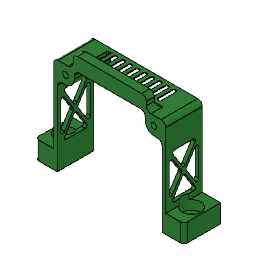
RM Carriage Setup (Defensemen) (Autodesk Fusion 360 archive; units mm, degrees)
design "LGR RM Front Holder (Defensemen)"
Autodesk Fusion 360 part; units mm, degrees
(part 1 of 2)
sketch "Sketch1" plane through (0, 0, 0) normal (0, 0, 1) x (1, 0, 0)
  line L0 (28.55, 26.275) -> (30.55, 26.275)
  line L1 (30.55, 26.275) -> (30.55, -26.275)
  line L2 (30.55, -26.275) -> (28.55, -26.275)
  line L3 (28.55, -26.275) -> (28.55, 26.275)
  line L4 (-28.55, -26.275) -> (-30.55, -26.275)
  line L5 (-28.55, 26.275) -> (-28.55, -26.275)
  line L6 (-30.55, -26.275) -> (-30.55, 26.275)
  line L7 (-30.55, 26.275) -> (-28.55, 26.275)
  line L8 (-30.55, 26.275) -> (30.55, 26.275)
  line L9 (30.55, 26.275) -> (30.55, 28.275)
  line L10 (30.55, 28.275) -> (-30.55, 28.275)
  line L11 (-30.55, 28.275) -> (-30.55, 26.275)
  dimension "d1" = 2
  dimension "d2" = 52.55
  dimension "d4" = 26.275
  dimension "d5" = 2
  dimension "d6" = 52.55
  dimension "d7" = 57.1
  dimension "d8" = 28.55
  dimension "d9" = 2
  constraint horizontal L0
  constraint vertical L1
  constraint horizontal L2
  constraint vertical L3
  constraint horizontal L7
  constraint vertical L5
  constraint horizontal L4
  constraint vertical L6
  constraint horizontal L2.end L4.start
  constraint horizontal L8
  constraint vertical L9
  constraint horizontal L10
  constraint vertical L11
  constraint vertical L0.end L9.end
  measures "d1" distance of L1 L3
  measures "d2" distance of L0 L2
  measures "d4" distance of origin L0
  measures "d5" distance of L5 L6
  measures "d6" distance of L4 L7
  measures "d7" distance of L3 L5
  measures "d8" distance of origin L5
  measures "d9" distance of L8 L10
extrude "Extrude1" add sketch "Sketch1" along normal blind 20
sketch "Sketch2" plane through (0, 0, 20) normal (0, 0, 1) x (-1, 0, 0)
  line L0 (-30.55, 26.275) -> (-30.55, -28.275)
  line L1 (-30.55, -28.275) -> (30.55, -28.275)
  line L2 (30.55, -28.275) -> (30.55, 26.275)
  line L3 (30.55, 26.275) -> (28.55, 26.275)
  line L4 (28.55, 26.275) -> (28.55, -26.275)
  line L5 (28.55, -26.275) -> (-28.55, -26.275)
  line L6 (-28.55, -26.275) -> (-28.55, 26.275)
  line L7 (-28.55, 26.275) -> (-30.55, 26.275)
  line L8 (-30.55, 26.275) -> (-40.55, 26.275)
  line L9 (-40.55, 26.275) -> (-40.55, 16.275)
  line L10 (-40.55, 16.275) -> (-30.55, 16.275)
  line L11 (-30.55, 16.275) -> (-30.55, 26.275)
  line L12 (30.55, 26.275) -> (40.55, 26.275)
  line L13 (40.55, 26.275) -> (40.55, 16.275)
  line L14 (40.55, 16.275) -> (30.55, 16.275)
  line L15 (30.55, 16.275) -> (30.55, 26.275)
  dimension "d12" = 10
  dimension "d13" = 10
  dimension "d14" = 10
  dimension "d15" = 10
  constraint horizontal L8
  constraint vertical L9
  constraint horizontal L10
  constraint vertical L11
  constraint coincident L0.start L7.end
  constraint horizontal L12
  constraint vertical L13
  constraint horizontal L14
  constraint vertical L15
  constraint coincident L2.end L3.start
  measures "d12" distance of L8 L10
  measures "d13" distance of L9 L11
  measures "d14" distance of L12 L14
  measures "d15" distance of L13 L15
extrude "Extrude2" add sketch "Sketch2" against normal blind 20 contours L0 L8 L9 L10 L11 | L2 L12 L13 L14 L15
fillet "Fillet1" radius 2 2 edges at (40.55, -21.275, 0) (-40.55, -21.275, 0)
sketch "Sketch3" plane through (0, -16.275, 0) normal (0, 1, 0) x (-1, 0, 0)
  arc A0 (38.55, 0) -> (40.55, 2) centre (38.55, 2) ccw
  line L0 (40.55, 2) -> (40.55, 20)
  line L1 (40.55, 20) -> (30.55, 20)
  line L2 (30.55, 20) -> (30.55, 0)
  line L3 (30.55, 0) -> (38.55, 0)
  point P0 (34.75, 10)
  point P1 (-34.75, 10)
  dimension "d20" = 5.8
  dimension "d21" = 10
  dimension "d22" = 69.5
  constraint horizontal P0 P1
  measures "d20" distance of L0 P0
  measures "d21" distance of L3 P0
  measures "d22" distance of P0 P1
hole "Hole1" at (-34.75, -16.275, 10) at (34.75, -16.275, 10) direction (0, -1, 0) diameter 5.3 end through all counterbore diameter 10 counterbore depth 5
sketch "Sketch4" plane through (0, -16.275, 0) normal (0, 1, 0) x (-1, 0, 0)
  arc A0 (30.55, 7.2871) -> (30.55, 12.7129) centre (34.75, 10) ccw
  line L0 (30.55, 7.2871) -> (30.55, 0)
  line L1 (30.55, 0) -> (38.55, 0)
  arc A1 (38.55, 0) -> (40.55, 2) centre (38.55, 2) ccw
  line L2 (40.55, 2) -> (40.55, 20)
  line L3 (40.55, 20) -> (30.55, 20)
  line L4 (30.55, 20) -> (30.55, 12.7129)
  circle A2 centre (34.75, 10) radius 5
  circle A3 centre (-34.75, 10) radius 5
  dimension "d28" = 10
  dimension "d29" = 69.5
  constraint concentric A0 A2
  constraint coincident A0.end A2
  constraint horizontal A0.centre A3.centre
  measures "d28" diameter of A3
  measures "d29" distance of A0.centre A3.centre
extrude "Extrude3" cut sketch "Sketch4" along normal blind 7 contours A0 A2 | A3
sketch "Sketch5" plane through (0, 28.275, 0) normal (0, 1, 0) x (-1, 0, 0)
  line L0 (-30.55, 0) -> (30.55, 0)
  line L1 (30.55, 0) -> (30.55, 20)
  line L2 (30.55, 20) -> (-30.55, 20)
  line L3 (-30.55, 20) -> (-30.55, 0)
  line L4 (-20, 20) -> (20, 20)
  line L5 (20, 20) -> (20, 0)
  line L6 (20, 0) -> (-20, 0)
  line L7 (-20, 0) -> (-20, 20)
  dimension "d32" = 40
  dimension "d96" = 20
  constraint horizontal L4
  constraint vertical L5
  constraint horizontal L6
  constraint vertical L7
  constraint coincident L0 L5.end
  constraint coincident L2 L4.start
  measures "d32" distance of L5 L7
  measures "d96" distance of origin L7
extrude "Extrude4" add sketch "Sketch5" along normal blind 10 contours L0 L2 L4 L5 L6 L7
sketch "Sketch6" plane through (0, 0, 0) normal (0, 0, -1) x (1, 0, 0)
  line L0 (20, -38.275) -> (20, -28.275)
  line L1 (-30.55, -28.275) -> (-20, -28.275)
  line L2 (30.55, -28.275) -> (30.55, 16.275)
  line L3 (30.55, 16.275) -> (38.55, 16.275)
  line L4 (38.55, 16.275) -> (38.55, 26.275)
  line L5 (38.55, 26.275) -> (28.55, 26.275)
  line L6 (28.55, 26.275) -> (28.55, -26.275)
  line L7 (28.55, -26.275) -> (-28.55, -26.275)
  line L8 (-28.55, -26.275) -> (-28.55, 26.275)
  line L9 (-28.55, 26.275) -> (-38.55, 26.275)
  line L10 (-38.55, 26.275) -> (-38.55, 16.275)
  line L11 (-38.55, 16.275) -> (-30.55, 16.275)
  line L12 (-30.55, 16.275) -> (-30.55, -28.275)
  line L13 (-20, -28.275) -> (-20, -38.275)
  line L14 (-20, -38.275) -> (20, -38.275)
  line L15 (-28.55, -26.275) -> (-19.3, -26.275)
  line L16 (-19.3, -23.775) -> (-19.3, -22.025)
  line L17 (-24.3, -17.025) -> (-26.05, -17.025)
  line L18 (-28.55, -17.025) -> (-28.55, -26.275)
  line L19 (28.55, -26.275) -> (19.3, -26.275)
  line L20 (19.3, -23.775) -> (19.3, -22.025)
  line L21 (24.3, -17.025) -> (26.05, -17.025)
  line L22 (28.55, -17.025) -> (28.55, -26.275)
  arc A0 (-19.3, -22.025) -> (-24.3, -17.025) centre (-24.3, -22.025) ccw
  arc A1 (24.3, -17.025) -> (19.3, -22.025) centre (24.3, -22.025) ccw
  line L23 (28.55, -14.525) -> (28.55, -10)
  line L24 (-28.55, -14.525) -> (-28.55, -10)
  arc A2 (26.05, -17.025) -> (28.55, -14.525) centre (26.05, -14.525) ccw
  arc A3 (-28.55, -14.525) -> (-26.05, -17.025) centre (-26.05, -14.525) ccw
  line L25 (16.8, -26.275) -> (13, -26.275)
  line L26 (-16.8, -26.275) -> (-13, -26.275)
  arc A4 (16.8, -26.275) -> (19.3, -23.775) centre (16.8, -23.775) ccw
  arc A5 (-19.3, -23.775) -> (-16.8, -26.275) centre (-16.8, -23.775) ccw
  line L27 (20, -28.275) -> (30.55, -28.275)
  dimension "d38" = 9.25
  dimension "d39" = 9.25
  dimension "d40" = 9.25
  dimension "d41" = 9.25
  dimension "d42" = 5
  dimension "d43" = 5
  dimension "d44" = 2.5
  dimension "d45" = 2.5
  dimension "d46" = 2.5
  dimension "d47" = 2.5
  constraint horizontal L15
  constraint vertical L16
  constraint horizontal L17
  constraint vertical L18
  constraint coincident L7.end L8.start
  constraint horizontal L19
  constraint vertical L20
  constraint horizontal L21
  constraint vertical L22
  constraint coincident L6.end L7.start
  constraint tangent L17 A0
  constraint tangent L16 A0
  constraint tangent L21 A1
  constraint tangent L20 A1
  constraint coincident L6 L23.end
  constraint coincident L8 L24.end
  constraint coincident L22.start L21
  constraint coincident L22.start L23
  constraint tangent L21 A2
  constraint tangent L23 A2
  constraint coincident L18.start L24
  constraint coincident L18.start L17
  constraint tangent L24 A3
  constraint tangent L17 A3
  constraint coincident L7 L25.end
  constraint coincident L7 L26.end
  constraint coincident L19.end L25
  constraint coincident L19.end L20
  constraint tangent L25 A4
  constraint tangent L20 A4
  constraint coincident L15.end L26
  constraint coincident L15.end L16
  constraint tangent L26 A5
  constraint tangent L16 A5
  measures "d38" distance of L16 L18
  measures "d39" distance of L15 L17
  measures "d40" distance of L20 L22
  measures "d41" distance of L19 L21
  measures "d42" radius of A0
  measures "d43" radius of A1
  measures "d44" radius of A2
  measures "d45" radius of A3
  measures "d46" radius of A4
  measures "d47" radius of A5
extrude "Extrude5" add sketch "Sketch6" against normal blind 20 contours L6 L7 L19 L20 L21 L22 A1 A2 A4 | L7 L8 L15 L16 L17 L18 A0 A3 A5
sketch "Sketch7" plane through (0, 0, 20) normal (0, 0, 1) x (-1, 0, 0)
  line L0 (-30.55, -28.275) -> (-20, -28.275)
  line L1 (-20, -28.275) -> (20, -28.275)
  line L2 (30.55, -28.275) -> (30.55, 16.275)
  line L3 (30.55, 16.275) -> (40.55, 16.275)
  line L4 (40.55, 16.275) -> (40.55, 26.275)
  line L5 (40.55, 26.275) -> (28.55, 26.275)
  line L6 (28.55, 26.275) -> (28.55, -14.525)
  arc A0 (26.05, -17.025) -> (28.55, -14.525) centre (26.05, -14.525) ccw
  line L7 (26.05, -17.025) -> (24.3, -17.025)
  arc A1 (24.3, -17.025) -> (19.3, -22.025) centre (24.3, -22.025) ccw
  line L8 (19.3, -22.025) -> (19.3, -23.775)
  arc A2 (16.8, -26.275) -> (19.3, -23.775) centre (16.8, -23.775) ccw
  line L9 (16.8, -26.275) -> (-16.8, -26.275)
  arc A3 (-19.3, -23.775) -> (-16.8, -26.275) centre (-16.8, -23.775) ccw
  line L10 (-19.3, -23.775) -> (-19.3, -22.025)
  arc A4 (-19.3, -22.025) -> (-24.3, -17.025) centre (-24.3, -22.025) ccw
  line L11 (-24.3, -17.025) -> (-26.05, -17.025)
  arc A5 (-28.55, -14.525) -> (-26.05, -17.025) centre (-26.05, -14.525) ccw
  line L12 (-28.55, -14.525) -> (-28.55, 26.275)
  line L13 (-28.55, 26.275) -> (-40.55, 26.275)
  line L14 (-40.55, 26.275) -> (-40.55, 16.275)
  line L15 (-40.55, 16.275) -> (-30.55, 16.275)
  line L16 (-30.55, 16.275) -> (-30.55, -28.275)
  line L17 (20, -28.275) -> (30.55, -28.275)
  point P0 (24.05, -21.775)
  point P1 (-24.05, -21.775)
  dimension "d52" = 6.5
  dimension "d54" = 6.5
  constraint horizontal P0 P1
  measures "d52" distance of L2 P0
  measures "d54" distance of L16 P1
hole "Hole2" at (-24.05, 21.775, 20) at (24.05, 21.775, 20) direction (0, 0, -1) diameter 3 end through all
sketch "Sketch10" plane through (-30.55, 0, 0) normal (-1, 0, 0) x (0, -1, 0)
  line L0 (-28.275, 0) -> (16.275, 0)
  line L1 (16.275, 0) -> (16.275, 7.2871)
  line L2 (16.275, 7.2871) -> (9.275, 7.2871)
  line L3 (9.275, 7.2871) -> (9.275, 12.7129)
  line L4 (9.275, 12.7129) -> (16.275, 12.7129)
  line L5 (16.275, 12.7129) -> (16.275, 20)
  line L6 (16.275, 20) -> (-28.275, 20)
  line L7 (-11.225, 15.2411) -> (-11.225, 4.8453)
  line L8 (13.275, 15.2453) -> (13.275, 4.8411)
  line L9 (-28.275, 20) -> (-28.275, 0)
  line L10 (-6.5475, 18) -> (8.5844, 18)
  line L11 (-6.5475, 2) -> (8.5844, 2)
  line L12 (-7.0853, 3.8431) -> (0.4635, 8.6578)
  line L13 (1.5372, 8.6589) -> (9.1204, 3.8442)
  line L14 (11.7503, 3.9899) -> (3.3712, 9.1548)
  line L15 (3.3657, 10.854) -> (11.7448, 16.0932)
  line L16 (9.1204, 16.1558) -> (1.5372, 11.3411)
  line L17 (0.4635, 11.3422) -> (-7.0853, 16.1569)
  line L18 (-9.6931, 16.0879) -> (-1.358, 10.8529)
  line L19 (-1.3634, 9.1558) -> (-9.6986, 3.9951)
  arc A0 (-9.6931, 16.0879) -> (-11.225, 15.2411) centre (-10.225, 15.2411) ccw
  arc A1 (-11.225, 4.8453) -> (-9.6986, 3.9951) centre (-10.225, 4.8453) ccw
  arc A2 (-1.3634, 9.1558) -> (-1.358, 10.8529) centre (-1.8898, 10.0061) ccw
  arc A3 (1.5372, 8.6589) -> (0.4635, 8.6578) centre (1.0012, 7.8147) ccw
  arc A4 (8.5844, 2) -> (9.1204, 3.8442) centre (8.5844, 3) ccw
  arc A5 (-7.0853, 3.8431) -> (-6.5475, 2) centre (-6.5475, 3) ccw
  arc A6 (11.7503, 3.9899) -> (13.275, 4.8411) centre (12.275, 4.8411) ccw
  arc A7 (13.275, 15.2453) -> (11.7448, 16.0932) centre (12.275, 15.2453) ccw
  arc A8 (9.1204, 16.1558) -> (8.5844, 18) centre (8.5844, 17) ccw
  arc A9 (-6.5475, 18) -> (-7.0853, 16.1569) centre (-6.5475, 17) ccw
  arc A10 (0.4635, 11.3422) -> (1.5372, 11.3411) centre (1.0012, 12.1853) ccw
  arc A11 (3.3657, 10.854) -> (3.3712, 9.1548) centre (3.8959, 10.0061) ccw
  line L20 (-28.275, 20) -> (-28.275, 0)
  point P0 (-11.225, 17.05)
  point P1 (-11.225, 3.05)
  point P2 (13.275, 17.05)
  point P3 (13.275, 3.05)
  point P4 (-9.975, 18)
  point P5 (12.025, 18)
  point P6 (-9.975, 2)
  point P7 (12.025, 2)
  point P8 (1.025, 10.05)
  point P9 (1, 9)
  point P10 (0, 10)
  point P11 (1, 11)
  point P12 (2, 10)
  dimension "d77" = 3
  dimension "d78" = 17.05
  dimension "d79" = 2
  dimension "d80" = 2
  dimension "d81" = 11
  dimension "d82" = 7
  dimension "d83" = 22
  dimension "d84" = 22
  dimension "d85" = 14
  dimension "d86" = 14
  dimension "d87" = 4.25
  dimension "d88" = 3.05
  dimension "d89" = 1
  constraint perpendicular L6 L7
  constraint vertical L8
  constraint horizontal L10
  constraint perpendicular L7 L11
  constraint horizontal P0 P2
  constraint vertical P4 P6
  constraint coincident P0 L18
  constraint coincident P0 L7
  constraint tangent L18 A0
  constraint tangent L7 A0
  constraint coincident P1 L7
  constraint coincident P1 L19
  constraint tangent L7 A1
  constraint tangent L19 A1
  constraint equal A0 A1
  constraint tangent L19 A2
  constraint tangent L18 A2
  constraint equal A0 A2
  constraint tangent L12 A3
  constraint tangent L13 A3
  constraint equal A0 A3
  constraint coincident P7 L13
  constraint coincident P7 L11
  constraint tangent L13 A4
  constraint tangent L11 A4
  constraint equal A0 A4
  constraint coincident P6 L11
  constraint coincident P6 L12
  constraint tangent L11 A5
  constraint tangent L12 A5
  constraint equal A0 A5
  constraint coincident P3 L14
  constraint coincident P3 L8
  constraint tangent L14 A6
  constraint tangent L8 A6
  constraint equal A0 A6
  constraint coincident P2 L8
  constraint coincident P2 L15
  constraint tangent L8 A7
  constraint tangent L15 A7
  constraint equal A0 A7
  constraint coincident P5 L16
  constraint coincident P5 L10
  constraint tangent L16 A8
  constraint tangent L10 A8
  constraint equal A0 A8
  constraint coincident P4 L17
  constraint coincident P4 L10
  constraint tangent L17 A9
  constraint tangent L10 A9
  constraint equal A0 A9
  constraint tangent L16 A10
  constraint tangent L17 A10
  constraint equal A0 A10
  constraint tangent L14 A11
  constraint tangent L15 A11
  constraint equal A0 A11
  measures "d77" distance of L5 L8
  measures "d78" distance of L7 L9
  measures "d79" distance of L6 L10
  measures "d80" distance of L0 L11
  measures "d81" horizontal distance of P5 P8
  measures "d82" vertical distance of P2 P8
  measures "d83" distance of P4 P5
  measures "d84" distance of P6 P7
  measures "d85" distance of P2 P3
  measures "d86" distance of P0 P1
  measures "d87" distance of L5 P5
  measures "d88" distance of L0 P3
  measures "d89" radius of A0
extrude "Extrude8" cut sketch "Sketch10" against normal blind 65 contours L2 L3 L4 L8 L14 L15 A6 A7 A11 | L2 L3 L4 L8 | L7 L18 L19 A0 A1 A2 | L10 L16 L17 A8 A9 A10 | L11 L12 L13 A3 A4 A5
extrude "Extrude9" cut 2 faces at (27.0333, 28.275, 6.6667) (-23.5167, 28.275, 13.3333) along direction (0, -1, 0) blind 1.55
extrude "Extrude10" cut 1 faces at (-6.6667, 38.275, 13.3333) along direction (0, -1, 0) blind 4.5
fillet "Fillet4" radius 2.5 6 edges at (-20, 26.725, 10) (-20, 33.775, 10) (-30.55, 26.725, 10) (20, 33.775, 10) (20, 26.725, 10) (30.55, 26.725, 10)
sketch "Sketch11" plane through (0, 33.775, 0) normal (0, 1, 0) x (-1, 0, 0)
  line L0 (-17.5, 20) -> (-17.5, 0)
  line L1 (-17.5, 0) -> (17.5, 0)
  line L2 (17.5, 0) -> (17.5, 20)
  line L3 (17.5, 20) -> (-17.5, 20)
  line L4 (-22.5, 4.5) -> (22.5, 4.5)
  line L5 (22.5, 4.5) -> (22.5, 20)
  line L6 (22.5, 20) -> (-22.5, 20)
  line L7 (-22.5, 20) -> (-22.5, 4.5)
  dimension "d99" = 4.5
  dimension "d100" = 45
  dimension "d101" = 15.5
  dimension "d102" = 22.5
  constraint horizontal L4
  constraint vertical L5
  constraint horizontal L6
  constraint vertical L7
  measures "d99" distance of L1 L4
  measures "d100" distance of L5 L7
  measures "d101" distance of L4 L6
  measures "d102" distance of origin L7
extrude "Extrude11" cut sketch "Sketch11" against normal blind 7.05 contours L0 L2 L3 L4 L6 | L0 L4 L6 L7 | L2 L4 L5 L6
fillet "Fillet7" radius 2 1 edges at (0, 26.725, 4.5)
sketch "Sketch14" plane through (0, 26.725, 0) normal (0, 1, 0) x (-1, 0, 0)
  line L0 (-22.5, 0) -> (-22.5, 6.5)
  line L1 (-22.5, 6.5) -> (22.5, 6.5)
  line L2 (22.5, 6.5) -> (22.5, 0)
  line L3 (22.5, 0) -> (28.05, 0)
  line L4 (28.05, 0) -> (28.05, 20)
  line L5 (28.05, 20) -> (-28.05, 20)
  line L6 (-28.05, 20) -> (-28.05, 0)
  line L7 (-28.05, 0) -> (-22.5, 0)
  line L8 (9.5, 8.5) -> (10.5, 8.5)
  line L9 (11, 9) -> (11, 17.5)
  line L10 (10.5, 18) -> (9.5, 18)
  line L11 (9, 17.5) -> (9, 9)
  line L12 (6.5, 18) -> (5.5, 18)
  line L13 (5, 17.5) -> (5, 9)
  line L14 (7, 9) -> (7, 17.5)
  line L15 (5.5, 8.5) -> (6.5, 8.5)
  line L16 (2.5, 18) -> (1.5, 18)
  line L17 (1, 17.5) -> (1, 9)
  line L18 (3, 9) -> (3, 17.5)
  line L19 (1.5, 8.5) -> (2.5, 8.5)
  line L20 (-1.5, 18) -> (-2.5, 18)
  line L21 (-3, 17.5) -> (-3, 9)
  line L22 (-1, 9) -> (-1, 17.5)
  line L23 (-2.5, 8.5) -> (-1.5, 8.5)
  line L24 (-5.5, 18) -> (-6.5, 18)
  line L25 (-7, 17.5) -> (-7, 9)
  line L26 (-5, 9) -> (-5, 17.5)
  line L27 (-6.5, 8.5) -> (-5.5, 8.5)
  line L28 (-9.5, 8.5) -> (-10.5, 8.5)
  line L29 (-11, 9) -> (-11, 17.5)
  line L30 (-10.5, 18) -> (-9.5, 18)
  line L31 (-9, 17.5) -> (-9, 9)
  arc A0 (10.5, 8.5) -> (11, 9) centre (10.5, 9) ccw
  arc A1 (11, 17.5) -> (10.5, 18) centre (10.5, 17.5) ccw
  arc A2 (9.5, 18) -> (9, 17.5) centre (9.5, 17.5) ccw
  arc A3 (9, 9) -> (9.5, 8.5) centre (9.5, 9) ccw
  arc A4 (6.5, 8.5) -> (7, 9) centre (6.5, 9) ccw
  arc A5 (5, 9) -> (5.5, 8.5) centre (5.5, 9) ccw
  arc A6 (5.5, 18) -> (5, 17.5) centre (5.5, 17.5) ccw
  arc A7 (7, 17.5) -> (6.5, 18) centre (6.5, 17.5) ccw
  arc A8 (2.5, 8.5) -> (3, 9) centre (2.5, 9) ccw
  arc A9 (1, 9) -> (1.5, 8.5) centre (1.5, 9) ccw
  arc A10 (1.5, 18) -> (1, 17.5) centre (1.5, 17.5) ccw
  arc A11 (3, 17.5) -> (2.5, 18) centre (2.5, 17.5) ccw
  arc A12 (-1.5, 8.5) -> (-1, 9) centre (-1.5, 9) ccw
  arc A13 (-3, 9) -> (-2.5, 8.5) centre (-2.5, 9) ccw
  arc A14 (-2.5, 18) -> (-3, 17.5) centre (-2.5, 17.5) ccw
  arc A15 (-1, 17.5) -> (-1.5, 18) centre (-1.5, 17.5) ccw
  arc A16 (-5.5, 8.5) -> (-5, 9) centre (-5.5, 9) ccw
  arc A17 (-7, 9) -> (-6.5, 8.5) centre (-6.5, 9) ccw
  arc A18 (-6.5, 18) -> (-7, 17.5) centre (-6.5, 17.5) ccw
  arc A19 (-5, 17.5) -> (-5.5, 18) centre (-5.5, 17.5) ccw
  arc A20 (-9.5, 8.5) -> (-9, 9) centre (-9.5, 9) ccw
  arc A21 (-11, 9) -> (-10.5, 8.5) centre (-10.5, 9) ccw
  arc A22 (-10.5, 18) -> (-11, 17.5) centre (-10.5, 17.5) ccw
  arc A23 (-9, 17.5) -> (-9.5, 18) centre (-9.5, 17.5) ccw
  line L32 (13, 17.5) -> (13, 9)
  arc A24 (13.5, 18) -> (13, 17.5) centre (13.5, 17.5) ccw
  arc A25 (13, 9) -> (13.5, 8.5) centre (13.5, 9) ccw
  arc A26 (14.5, 8.5) -> (15, 9) centre (14.5, 9) ccw
  line L33 (13.5, 8.5) -> (14.5, 8.5)
  line L34 (15, 9) -> (15, 17.5)
  line L35 (14.5, 18) -> (13.5, 18)
  arc A27 (15, 17.5) -> (14.5, 18) centre (14.5, 17.5) ccw
  line L36 (17, 17.5) -> (17, 9)
  arc A28 (17.5, 18) -> (17, 17.5) centre (17.5, 17.5) ccw
  arc A29 (17, 9) -> (17.5, 8.5) centre (17.5, 9) ccw
  arc A30 (18.5, 8.5) -> (19, 9) centre (18.5, 9) ccw
  line L37 (17.5, 8.5) -> (18.5, 8.5)
  line L38 (19, 9) -> (19, 17.5)
  line L39 (18.5, 18) -> (17.5, 18)
  arc A31 (19, 17.5) -> (18.5, 18) centre (18.5, 17.5) ccw
  line L40 (-15, 17.5) -> (-15, 9)
  arc A32 (-14.5, 18) -> (-15, 17.5) centre (-14.5, 17.5) ccw
  arc A33 (-15, 9) -> (-14.5, 8.5) centre (-14.5, 9) ccw
  arc A34 (-13.5, 8.5) -> (-13, 9) centre (-13.5, 9) ccw
  line L41 (-14.5, 8.5) -> (-13.5, 8.5)
  line L42 (-13, 9) -> (-13, 17.5)
  line L43 (-13.5, 18) -> (-14.5, 18)
  arc A35 (-13, 17.5) -> (-13.5, 18) centre (-13.5, 17.5) ccw
  line L44 (-19, 17.5) -> (-19, 9)
  arc A36 (-18.5, 18) -> (-19, 17.5) centre (-18.5, 17.5) ccw
  arc A37 (-19, 9) -> (-18.5, 8.5) centre (-18.5, 9) ccw
  arc A38 (-17.5, 8.5) -> (-17, 9) centre (-17.5, 9) ccw
  line L45 (-18.5, 8.5) -> (-17.5, 8.5)
  line L46 (-17, 9) -> (-17, 17.5)
  line L47 (-17.5, 18) -> (-18.5, 18)
  arc A39 (-17, 17.5) -> (-17.5, 18) centre (-17.5, 17.5) ccw
  dimension "d115" = 2
  dimension "d116" = 2
  dimension "d117" = 2
  dimension "d118" = 2
  dimension "d119" = 2
  dimension "d120" = 2
  dimension "d121" = 2
  dimension "d122" = 2
  dimension "d123" = 2
  dimension "d125" = 2
  dimension "d127" = 2
  dimension "d128" = 2
  dimension "d129" = 2
  dimension "d130" = 2
  dimension "d131" = 2
  dimension "d132" = 2
  dimension "d133" = 2
  dimension "d134" = 2
  dimension "d135" = 2
  dimension "d136" = 2
  dimension "d137" = 2
  dimension "d138" = 2
  dimension "d139" = 2
  dimension "d140" = 1
  dimension "d141" = 0.5
  dimension "d144" = 2
  dimension "d145" = 0.5
  dimension "d146" = 2
  dimension "d147" = 0.5
  dimension "d148" = 2
  dimension "d149" = 0.5
  dimension "d150" = 2
  dimension "d151" = 0.5
  dimension "d152" = 2
  dimension "d153" = 2
  dimension "d154" = 2
  dimension "d155" = 2
  dimension "d156" = 2
  dimension "d157" = 2
  dimension "d158" = 2
  dimension "d159" = 2
  dimension "d160" = 2
  dimension "d161" = 2
  dimension "d162" = 2
  dimension "d163" = 2
  constraint horizontal L8
  constraint vertical L9
  constraint horizontal L10
  constraint vertical L11
  constraint horizontal L15
  constraint vertical L14
  constraint horizontal L12
  constraint vertical L13
  constraint horizontal L19
  constraint vertical L18
  constraint horizontal L16
  constraint vertical L17
  constraint horizontal L23
  constraint vertical L22
  constraint horizontal L20
  constraint vertical L21
  constraint horizontal L27
  constraint vertical L26
  constraint horizontal L24
  constraint vertical L25
  constraint horizontal L28
  constraint vertical L29
  constraint horizontal L30
  constraint vertical L31
  constraint tangent L8 A0
  constraint tangent L9 A0
  constraint tangent L9 A1
  constraint tangent L10 A1
  constraint equal A0 A1
  constraint tangent L10 A2
  constraint tangent L11 A2
  constraint equal A0 A2
  constraint tangent L11 A3
  constraint tangent L8 A3
  constraint equal A0 A3
  constraint tangent L14 A4
  constraint tangent L15 A4
  constraint equal A0 A4
  constraint tangent L15 A5
  constraint tangent L13 A5
  constraint equal A0 A5
  constraint tangent L13 A6
  constraint tangent L12 A6
  constraint equal A0 A6
  constraint tangent L12 A7
  constraint tangent L14 A7
  constraint equal A0 A7
  constraint tangent L18 A8
  constraint tangent L19 A8
  constraint equal A0 A8
  constraint tangent L19 A9
  constraint tangent L17 A9
  constraint equal A0 A9
  constraint tangent L17 A10
  constraint tangent L16 A10
  constraint equal A0 A10
  constraint tangent L16 A11
  constraint tangent L18 A11
  constraint equal A0 A11
  constraint tangent L22 A12
  constraint tangent L23 A12
  constraint equal A0 A12
  constraint tangent L23 A13
  constraint tangent L21 A13
  constraint equal A0 A13
  constraint tangent L21 A14
  constraint tangent L20 A14
  constraint equal A0 A14
  constraint tangent L20 A15
  constraint tangent L22 A15
  constraint equal A0 A15
  constraint tangent L26 A16
  constraint tangent L27 A16
  constraint equal A0 A16
  constraint tangent L27 A17
  constraint tangent L25 A17
  constraint equal A0 A17
  constraint tangent L25 A18
  constraint tangent L24 A18
  constraint equal A0 A18
  constraint tangent L24 A19
  constraint tangent L26 A19
  constraint equal A0 A19
  constraint tangent L31 A20
  constraint tangent L28 A20
  constraint equal A0 A20
  constraint tangent L28 A21
  constraint tangent L29 A21
  constraint equal A0 A21
  constraint tangent L29 A22
  constraint tangent L30 A22
  constraint equal A0 A22
  constraint tangent L30 A23
  constraint tangent L31 A23
  constraint equal A0 A23
  constraint horizontal L33
  constraint vertical L34
  constraint horizontal L35
  constraint vertical L32
  constraint tangent A26 L33
  constraint tangent A26 L34
  constraint tangent L34 A27
  constraint tangent L35 A27
  constraint equal A26 A27
  constraint tangent A24 L35
  constraint tangent L32 A24
  constraint equal A24 A26
  constraint tangent L32 A25
  constraint tangent A25 L33
  constraint equal A25 A26
  constraint horizontal L37
  constraint vertical L38
  constraint horizontal L39
  constraint vertical L36
  constraint tangent A30 L37
  constraint tangent A30 L38
  constraint tangent L38 A31
  constraint tangent L39 A31
  constraint equal A30 A31
  constraint tangent A28 L39
  constraint tangent L36 A28
  constraint equal A28 A30
  constraint tangent L36 A29
  constraint tangent A29 L37
  constraint equal A29 A30
  constraint horizontal L41
  constraint vertical L42
  constraint horizontal L43
  constraint vertical L40
  constraint tangent A34 L41
  constraint tangent A34 L42
  constraint tangent L42 A35
  constraint tangent L43 A35
  constraint equal A34 A35
  constraint tangent A32 L43
  constraint tangent L40 A32
  constraint equal A32 A34
  constraint tangent L40 A33
  constraint tangent A33 L41
  constraint equal A33 A34
  constraint horizontal L45
  constraint vertical L46
  constraint horizontal L47
  constraint vertical L44
  constraint tangent A38 L45
  constraint tangent A38 L46
  constraint tangent L46 A39
  constraint tangent L47 A39
  constraint equal A38 A39
  constraint tangent A36 L47
  constraint tangent L44 A36
  constraint equal A36 A38
  constraint tangent L44 A37
  constraint tangent A37 L45
  constraint equal A37 A38
  measures "d115" distance of L1 L8
  measures "d116" distance of L5 L10
  measures "d117" distance of L9 L11
  measures "d118" distance of L13 L14
  measures "d119" distance of L17 L18
  measures "d120" distance of L21 L22
  measures "d121" distance of L25 L26
  measures "d122" distance of L1 L19
  measures "d123" distance of L5 L16
  measures "d125" distance of L17 L22
  measures "d127" distance of L13 L18
  measures "d128" distance of L11 L14
  measures "d129" distance of L21 L26
  measures "d130" distance of L25 L31
  measures "d131" distance of L1 L15
  measures "d132" distance of L1 L23
  measures "d133" distance of L1 L27
  measures "d134" distance of L1 L28
  measures "d135" distance of L5 L30
  measures "d136" distance of L5 L24
  measures "d137" distance of L5 L20
  measures "d138" distance of L5 L12
  measures "d139" distance of L29 L31
  measures "d140" distance of origin L17
  measures "d141" radius of A0
  measures "d144" distance of L32 L34
  measures "d145" radius of A26
  measures "d146" distance of L36 L38
  measures "d147" radius of A30
  measures "d148" distance of L40 L42
  measures "d149" radius of A34
  measures "d150" distance of L44 L46
  measures "d151" radius of A38
  measures "d152" distance of L9 L32
  measures "d153" distance of L34 L36
  measures "d154" distance of L5 L35
  measures "d155" distance of L5 L39
  measures "d156" distance of L1 L33
  measures "d157" distance of L1 L37
  measures "d158" distance of L29 L42
  measures "d159" distance of L40 L46
  measures "d160" distance of L5 L47
  measures "d161" distance of L5 L43
  measures "d162" distance of L1 L41
  measures "d163" distance of L1 A38.start
extrude "Extrude14" cut sketch "Sketch14" against normal blind 5 contours L8 L9 L10 L11 A0 A1 A2 A3 | L12 L13 L14 L15 A4 A5 A6 A7 | L16 L17 L18 L19 A8 A9 A10 A11 | L20 L21 L22 L23 A12 A13 A14 A15 | L24 L25 L26 L27 A16 A17 A18 A19 | L28 L29 L30 L31 A20 A21 A22 A23 | L32 A24 A25 A26 L33 L34 L35 A27 | L36 A28 A29 A30 L37 L38 L39 A31 | L40 A32 A33 A34 L41 L42 L43 A35 | L44 A36 A37 A38 L45 L46 L47 A39
equation "d4 = ( 52.55 / 2 ) * 1 mm"
equation "d8 = ( 57.1 / 2 ) * 1 mm"
equation "d20 = 3.75 mm + 2.5 mm - 0.45 mm"
equation "d88 = ( ( 20.1 - 14 ) / 2 ) * 1 mm"
equation "d102 = ( 45 / 2 ) * 1 mm"

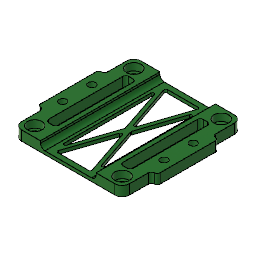
design "LGR RM Carriage Bracket (Defensemen)"
Autodesk Fusion 360 part; units mm, degrees
sketch "Sketch1" plane through (0, 0, 0) normal (0, 0, 1) x (1, 0, 0)
  line L0 (-41, 41) -> (41, 41)
  line L1 (41, 41) -> (41, -41)
  line L2 (41, -41) -> (-41, -41)
  line L3 (-41, -41) -> (-41, 41)
  dimension "d1" = 82
  dimension "d2" = 82
  dimension "d3" = 41
  dimension "d4" = 41
  constraint horizontal L0
  constraint vertical L1
  constraint horizontal L2
  constraint vertical L3
  measures "d1" distance of L1 L3
  measures "d2" distance of L0 L2
  measures "d3" distance of origin L1
  measures "d4" distance of origin L0
extrude "Extrude1" add sketch "Sketch1" along normal blind 6.5
sketch "Sketch2" plane through (0, 0, 6.5) normal (0, 0, 1) x (-1, 0, 0)
  line L0 (41, 41) -> (-41, 41)
  line L1 (-41, 41) -> (-41, -41)
  line L2 (-41, -41) -> (41, -41)
  line L3 (41, -41) -> (41, 41)
  point P0 (34, -30)
  point P1 (-34, -30)
  point P2 (-34, 30)
  point P3 (34, 30)
  dimension "d7" = 68
  dimension "d8" = 60
  dimension "d9" = 7
  dimension "d10" = 11
  constraint horizontal P0 P1
  constraint vertical P1 P2
  constraint horizontal P2 P3
  constraint vertical P0 P3
  measures "d7" distance of P0 P1
  measures "d8" distance of P1 P2
  measures "d9" distance of L1 P1
  measures "d10" distance of L2 P1
hole "Hole1" at (-34, 30, 6.5) at (34, 30, 6.5) at (34, -30, 6.5) at (-34, -30, 6.5) direction (0, 0, -1) diameter 5.5 depth 10 tip angle 180 counterbore diameter 10 counterbore depth 5
sketch "Sketch3" plane through (0, 0, 6.5) normal (0, 0, 1) x (-1, 0, 0)
  circle A0 centre (-34, 30) radius 5
  circle A1 centre (34, -30) radius 5
  circle A2 centre (-34, -30) radius 5
  circle A3 centre (34, 30) radius 5
  line L0 (41, 41) -> (-41, 41)
  line L1 (-41, 41) -> (-41, -41)
  line L2 (-41, -41) -> (41, -41)
  line L3 (41, -41) -> (41, 41)
  line L4 (41, -19.05) -> (-41, -19.05)
  line L5 (-41, -19.05) -> (-41, 19.05)
  line L6 (-41, 19.05) -> (41, 19.05)
  line L7 (41, 19.05) -> (41, -19.05)
  dimension "d16" = 38.1
  dimension "d17" = 19.05
  constraint horizontal L4
  constraint vertical L5
  constraint horizontal L6
  constraint vertical L7
  constraint coincident L1 L5.end
  constraint coincident L3 L4.start
  measures "d16" distance of L4 L6
  measures "d17" distance of origin L6
extrude "Extrude2" cut sketch "Sketch3" against normal blind 4.5 contours L1 L3 L4 L5 L6 L7
fillet "Fillet1" radius 3 2 edges at (0, 19.05, 2) (0, -19.05, 2)
sketch "Sketch4" plane through (0, 0, 6.5) normal (0, 0, 1) x (-1, 0, 0)
  line L0 (41, -19.05) -> (-41, -19.05)
  line L1 (-41, -19.05) -> (-41, -41)
  line L2 (-41, -41) -> (41, -41)
  line L3 (41, -41) -> (41, -19.05)
  circle A0 centre (34, -30) radius 5
  circle A1 centre (-34, -30) radius 5
  line L4 (41, 41) -> (-41, 41)
  line L5 (41, 19.05) -> (41, 41)
  point P0 (-10, -34.75)
  point P1 (10, -34.75)
  point P2 (-10, 34.75)
  point P3 (10, 34.75)
  point P4 (-5.7919, 53.9874)
  dimension "d23" = 6.25
  dimension "d24" = 6.25
  dimension "d25" = 20
  dimension "d26" = 31
  constraint vertical P0 P2
  constraint horizontal P2 P3
  constraint vertical P1 P3
  constraint horizontal P0 P1
  measures "d23" distance of P2 L4
  measures "d24" distance of L2 P0
  measures "d25" distance of P0 P1
  measures "d26" distance of P3 L5
hole "Hole2" at (10, 34.75, 6.5) at (-10, 34.75, 6.5) at (10, -34.75, 6.5) at (-10, -34.75, 6.5) direction (0, 0, -1) diameter 5 end through all
sketch "Sketch7" plane through (0, 0, 6.5) normal (0, 0, 1) x (-1, 0, 0)
  circle A0 centre (-10, 34.75) radius 2.5
  circle A1 centre (10, 34.75) radius 2.5
  line L0 (-41, 19.05) -> (41, 19.05)
  line L1 (41, 19.05) -> (41, 41)
  line L2 (41, 41) -> (-41, 41)
  line L3 (-41, 41) -> (-41, 19.05)
  circle A2 centre (34, 30) radius 5
  circle A3 centre (-34, 30) radius 5
  line L4 (25.5, 22.05) -> (-25.5, 22.05)
  line L5 (-27.5, 24.05) -> (-27.5, 27.05)
  line L6 (-25.5, 29.05) -> (25.5, 29.05)
  line L7 (27.5, 27.05) -> (27.5, 24.05)
  line L8 (25.5, -29.05) -> (-25.5, -29.05)
  line L9 (-27.5, -27.05) -> (-27.5, -24.05)
  line L10 (-25.5, -22.05) -> (25.5, -22.05)
  line L11 (27.5, -24.05) -> (27.5, -27.05)
  line L12 (41, -19.05) -> (-41, -19.05)
  line L13 (-41, -19.05) -> (-41, -41)
  arc A4 (25.5, -29.05) -> (27.5, -27.05) centre (25.5, -27.05) ccw
  arc A5 (27.5, -24.05) -> (25.5, -22.05) centre (25.5, -24.05) ccw
  arc A6 (-25.5, -22.05) -> (-27.5, -24.05) centre (-25.5, -24.05) ccw
  arc A7 (-27.5, -27.05) -> (-25.5, -29.05) centre (-25.5, -27.05) ccw
  arc A8 (25.5, 22.05) -> (27.5, 24.05) centre (25.5, 24.05) ccw
  arc A9 (27.5, 27.05) -> (25.5, 29.05) centre (25.5, 27.05) ccw
  arc A10 (-25.5, 29.05) -> (-27.5, 27.05) centre (-25.5, 27.05) ccw
  arc A11 (-27.5, 24.05) -> (-25.5, 22.05) centre (-25.5, 24.05) ccw
  dimension "d31" = 55
  dimension "d32" = 7
  dimension "d33" = 3
  dimension "d34" = 13.5
  dimension "d35" = 7
  dimension "d36" = 3
  dimension "d37" = 13.5
  dimension "d38" = 55
  dimension "d39" = 2
  constraint horizontal L4
  constraint vertical L5
  constraint horizontal L6
  constraint vertical L7
  constraint horizontal L8
  constraint vertical L9
  constraint horizontal L10
  constraint vertical L11
  constraint tangent L8 A4
  constraint tangent L11 A4
  constraint tangent L11 A5
  constraint tangent L10 A5
  constraint equal A4 A5
  constraint tangent L10 A6
  constraint tangent L9 A6
  constraint equal A4 A6
  constraint tangent L9 A7
  constraint tangent L8 A7
  constraint equal A4 A7
  constraint tangent L4 A8
  constraint tangent L7 A8
  constraint equal A4 A8
  constraint tangent L7 A9
  constraint tangent L6 A9
  constraint equal A4 A9
  constraint tangent L6 A10
  constraint tangent L5 A10
  constraint equal A4 A10
  constraint tangent L5 A11
  constraint tangent L4 A11
  constraint equal A4 A11
  measures "d31" distance of L5 L7
  measures "d32" distance of L4 L6
  measures "d33" distance of L0 L4
  measures "d34" distance of L1 L7
  measures "d35" distance of L8 L10
  measures "d36" distance of L10 L12
  measures "d37" distance of L9 L13
  measures "d38" distance of L9 L11
  measures "d39" radius of A4
extrude "Extrude3" cut sketch "Sketch7" against normal blind 6.5 contours L4 L5 L6 L7 A8 A9 A10 A11 | L8 L9 L10 L11 A4 A5 A6 A7
ref_plane "WorkPlane1" through (0, 0, 6.5) normal (0, 0, -1) x (-1, 0, 0)
sketch "Sketch9" plane through (0, 0, 6.5) normal (0, 0, -1) x (-1, 0, 0)
  line L0 (41, 41) -> (21, 41)
  line L1 (21, 41) -> (21, 37)
  line L2 (21, 37) -> (41, 37)
  line L3 (41, 37) -> (41, 41)
  line L4 (-21, 41) -> (-41, 41)
  line L5 (-41, 41) -> (-41, 37)
  line L6 (-41, 37) -> (-21, 37)
  line L7 (-21, 37) -> (-21, 41)
  line L8 (41, -37) -> (21, -37)
  line L9 (21, -37) -> (21, -41)
  line L10 (21, -41) -> (41, -41)
  line L11 (41, -41) -> (41, -37)
  line L12 (-41, -41) -> (-21, -41)
  line L13 (-21, -41) -> (-21, -37)
  line L14 (-21, -37) -> (-41, -37)
  line L15 (-41, -37) -> (-41, -41)
  point P0 (41, 41)
  dimension "d59" = 82
  dimension "d60" = 82
  dimension "d61" = 4
  dimension "d62" = 20
  dimension "d63" = 20
  dimension "d64" = 4
  dimension "d65" = 20
  dimension "d66" = 20
  dimension "d67" = 4
  dimension "d68" = 4
  constraint horizontal L0
  constraint vertical L1
  constraint horizontal L2
  constraint vertical L3
  constraint horizontal L4
  constraint vertical L5
  constraint horizontal L6
  constraint vertical L7
  constraint horizontal L8
  constraint vertical L9
  constraint horizontal L10
  constraint vertical L11
  constraint horizontal L12
  constraint vertical L13
  constraint horizontal L14
  constraint vertical L15
  constraint vertical P0 L10.end
  constraint horizontal P0 L4.end
  constraint vertical L4.end L12.start
  constraint horizontal L10.end L12.start
  constraint vertical P0 L0.start
  constraint horizontal L0.end P0
  measures "d59" distance of L3 L5
  measures "d60" distance of L0 L10
  measures "d61" distance of L0 L2
  measures "d62" distance of L1 L3
  measures "d63" distance of L5 L7
  measures "d64" distance of L4 L6
  measures "d65" distance of L13 L15
  measures "d66" distance of L9 L11
  measures "d67" distance of L8 L10
  measures "d68" distance of L12 L14
extrude "Extrude5" cut sketch "Sketch9" along normal blind 6.5
fillet "Fillet2" radius 5 4 edges at (-41, 37, 3.25) (41, 37, 3.25) (41, -37, 3.25) (-41, -37, 3.25)
fillet "Fillet3" radius 2 8 edges at (-21, -41, 3.25) (-21, -37, 3.25) (21, -37, 3.25) (21, -41, 3.25) (21, 37, 3.25) (21, 41, 3.25) (-21, 41, 3.25) (-21, 37, 3.25)
sketch "Sketch10" plane through (0, 0, 2) normal (0, 0, 1) x (-1, 0, 0)
  line L0 (41, 16.05) -> (-41, 16.05)
  line L1 (-41, 16.05) -> (-41, -16.05)
  line L2 (-41, -16.05) -> (41, -16.05)
  line L3 (41, -16.05) -> (41, 16.05)
  line L4 (29.8377, -14) -> (-29.8377, -14)
  line L5 (29.8377, 14) -> (-29.8377, 14)
  line L6 (37.5, -10.6064) -> (37.5, 10.6064)
  line L7 (-37.5, -10.6064) -> (-37.5, 10.6064)
  line L8 (41, -19.05) -> (-41, -19.05)
  line L9 (30.154, 12.0513) -> (0.3162, 2.1054)
  line L10 (-0.3162, 2.1054) -> (-30.154, 12.0513)
  line L11 (-36.1798, 11.5537) -> (-4.8025, 0.9473)
  line L12 (-4.8025, -0.9473) -> (-36.1798, -11.5537)
  line L13 (-30.154, -12.0513) -> (-0.3162, -2.1054)
  line L14 (0.3162, -2.1054) -> (30.154, -12.0513)
  line L15 (36.1798, -11.5537) -> (4.8025, -0.9473)
  line L16 (4.8025, 0.9473) -> (36.1798, 11.5537)
  arc A0 (29.8377, -14) -> (30.154, -12.0513) centre (29.8377, -13) ccw
  arc A1 (0.3162, -2.1054) -> (-0.3162, -2.1054) centre (0, -3.0541) ccw
  arc A2 (-30.154, -12.0513) -> (-29.8377, -14) centre (-29.8377, -13) ccw
  arc A3 (-37.5, -10.6064) -> (-36.1798, -11.5537) centre (-36.5, -10.6064) ccw
  arc A4 (-36.1798, 11.5537) -> (-37.5, 10.6064) centre (-36.5, 10.6064) ccw
  arc A5 (-4.8025, -0.9473) -> (-4.8025, 0.9473) centre (-5.1228, 0) ccw
  arc A6 (-0.3162, 2.1054) -> (0.3162, 2.1054) centre (0, 3.0541) ccw
  arc A7 (-29.8377, 14) -> (-30.154, 12.0513) centre (-29.8377, 13) ccw
  arc A8 (30.154, 12.0513) -> (29.8377, 14) centre (29.8377, 13) ccw
  arc A9 (37.5, 10.6064) -> (36.1798, 11.5537) centre (36.5, 10.6064) ccw
  arc A10 (36.1798, -11.5537) -> (37.5, -10.6064) centre (36.5, -10.6064) ccw
  arc A11 (4.8025, 0.9473) -> (4.8025, -0.9473) centre (5.1228, 0) ccw
  point P0 (36, -14)
  point P1 (-36, -14)
  point P2 (-37.5, -12)
  point P3 (-37.5, 12)
  point P4 (0, -2)
  point P5 (-2, 0)
  point P6 (0, 2)
  point P7 (2, 0)
  dimension "d75" = 72
  dimension "d76" = 24
  dimension "d77" = 5
  dimension "d78" = 7.05
  dimension "d79" = 2.05
  dimension "d80" = 2.05
  dimension "d81" = 3.5
  dimension "d82" = 3.5
  dimension "d83" = 1
  constraint parallel L2 L4
  constraint perpendicular L3 L5
  constraint perpendicular L5 L6
  constraint perpendicular L4 L7
  constraint coincident P0 L4
  constraint coincident P0 L14
  constraint tangent L4 A0
  constraint tangent L14 A0
  constraint tangent L14 A1
  constraint tangent L13 A1
  constraint equal A0 A1
  constraint coincident P1 L13
  constraint coincident P1 L4
  constraint tangent L13 A2
  constraint tangent L4 A2
  constraint equal A0 A2
  constraint coincident P2 L12
  constraint coincident P2 L7
  constraint tangent L12 A3
  constraint tangent L7 A3
  constraint equal A0 A3
  constraint coincident P3 L7
  constraint coincident P3 L11
  constraint tangent L7 A4
  constraint tangent L11 A4
  constraint equal A0 A4
  constraint tangent L11 A5
  constraint tangent L12 A5
  constraint equal A0 A5
  constraint tangent L10 A6
  constraint tangent L9 A6
  constraint equal A0 A6
  constraint tangent L10 A7
  constraint tangent L5 A7
  constraint equal A0 A7
  constraint tangent L5 A8
  constraint tangent L9 A8
  constraint equal A0 A8
  constraint tangent L16 A9
  constraint tangent L6 A9
  constraint equal A0 A9
  constraint tangent L6 A10
  constraint tangent L15 A10
  constraint equal A0 A10
  constraint tangent L15 A11
  constraint tangent L16 A11
  constraint equal A0 A11
  measures "d75" distance of P0 P1
  measures "d76" distance of P2 P3
  measures "d77" distance of L1 P1
  measures "d78" distance of P2 L8
  measures "d79" distance of L2 L4
  measures "d80" distance of L0 L5
  measures "d81" distance of L1 L7
  measures "d82" distance of L3 L6
  measures "d83" radius of A0
extrude "Extrude6" cut sketch "Sketch10" against normal blind 2 contours L4 L13 L14 A0 A1 A2 | L5 L9 L10 A6 A7 A8 | L6 L15 L16 A9 A10 A11 | L7 L11 L12 A3 A4 A5
extrude "Extrude7" add 1 faces at (8.5, 16.6833, 0) along direction (0, 0, -1) blind 0.25
equation "d3 = ( 82 / 2 ) * 1 mm"
equation "d4 = ( 82 / 2 ) * 1 mm"
equation "d9 = ( ( 82 - 68 ) / 2 ) * 1 mm"
equation "d10 = ( ( 82 - 60 ) / 2 ) * 1 mm"
equation "d17 = ( 38.1 / 2 ) * 1 mm"
equation "d26 = ( ( 82 - 20 ) / 2 ) * 1 mm"
equation "d34 = ( ( 82 - 55 ) / 2 ) * 1 mm"
equation "d37 = ( ( 82 - 55 ) / 2 ) * 1 mm"
equation "d77 = ( ( 82 - 72 ) / 2 ) * 1 mm"
equation "d78 = ( ( 38.1 - 24 ) / 2 ) * 1 mm"

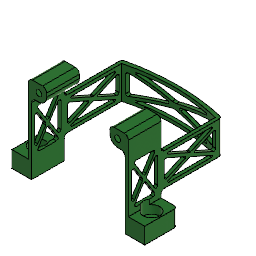
design "LGR RM Back Holder (Defensemen)"
Autodesk Fusion 360 part; units mm, degrees
sketch "Sketch1" plane through (0, 0, 0) normal (0, 0, 1) x (1, 0, 0)
  line L0 (-30.55, 55) -> (-28.55, 55)
  line L1 (-28.55, 55) -> (-28.55, 0)
  line L2 (-28.55, 0) -> (-30.55, 0)
  line L3 (-30.55, 0) -> (-30.55, 55)
  line L4 (28.55, 55) -> (30.55, 55)
  line L5 (30.55, 55) -> (30.55, 0)
  line L6 (30.55, 0) -> (28.55, 0)
  line L7 (28.55, 0) -> (28.55, 55)
  dimension "d1" = 55
  dimension "d2" = 55
  dimension "d3" = 2
  dimension "d4" = 2
  dimension "d5" = 57.1
  dimension "d6" = 28.55
  constraint horizontal L0
  constraint vertical L1
  constraint horizontal L2
  constraint vertical L3
  constraint horizontal L4
  constraint vertical L5
  constraint horizontal L6
  constraint vertical L7
  constraint horizontal L0.start L4.start
  constraint horizontal origin L1.end
  measures "d1" distance of L0 L2
  measures "d2" distance of L4 L6
  measures "d3" distance of L1 L3
  measures "d4" distance of L5 L7
  measures "d5" distance of L1 L7
  measures "d6" distance of origin L7
extrude "Extrude1" add sketch "Sketch1" along normal blind 20 makes body 1 at (-28.55, 36.6667, 6.6667) makes body 2 at (30.55, 36.6667, 6.6667)
sketch "Sketch3" plane through (0, 0, 20) normal (0, 0, 1) x (-1, 0, 0)
  line L0 (-28.55, 0) -> (-30.55, 0)
  line L1 (-30.55, 0) -> (-30.55, -55)
  line L2 (-30.55, -55) -> (-28.55, -55)
  line L3 (-28.55, -55) -> (-28.55, 0)
  arc A0 (-28.55, -55) -> (28.55, -55) centre (0, 53.299) ccw
  arc A1 (-30.55, -57) -> (30.55, -57) centre (0, 67.272) ccw
  line L4 (30.55, -57) -> (30.55, -55)
  line L5 (-30.55, -57) -> (-30.55, -55)
  line L6 (-28.55, -55) -> (-30.55, -55)
  line L7 (28.55, -55) -> (30.55, -55)
  point P0 (-28.55, -55)
  point P1 (28.55, -55)
  point P2 (0, -58.7)
  point P3 (0, -60.7)
  point P4 (30.55, -57)
  point P5 (-30.55, -57)
  point P6 (30.55, -55)
  point P7 (28.55, -55)
  dimension "d9" = 3.7
  dimension "d10" = 2
  dimension "d11" = 2
  dimension "d12" = 2
  constraint coincident P0 L2.end
  constraint coincident P2 A0
  constraint coincident P7 P1
  constraint vertical origin P2
  constraint vertical P2 P3
  constraint vertical L1.end P5
  constraint vertical P4 P6
  constraint coincident P3 A1
  constraint coincident P5 A1.start
  constraint coincident P4 A1.end
  constraint coincident P6 L4.end
  constraint coincident L1.end L2.start
  measures "d9" vertical distance of P0 P2
  measures "d10" distance of P2 P3
  measures "d11" distance of P4 P6
  measures "d12" distance of L1.end P5
extrude "Extrude2" add sketch "Sketch3" against normal blind 20 contours L2 A0 A1 L4 L5 L6 L7 bodies 1 2
sketch "Sketch4" plane through (30.55, 0, 0) normal (1, 0, 0) x (0, 1, 0)
  line L0 (0, 0) -> (57, 0)
  line L1 (57, 0) -> (57, 20)
  line L2 (57, 20) -> (0, 20)
  line L3 (0, 20) -> (0, 0)
  line L4 (0, 0) -> (20, 0)
  line L5 (20, 0) -> (20, -4)
  line L6 (20, -4) -> (0, -4)
  line L7 (0, -4) -> (0, 0)
  dimension "d15" = 4
  dimension "d16" = 20
  constraint horizontal L4
  constraint vertical L5
  constraint horizontal L6
  constraint vertical L7
  constraint coincident L0.start L3.end
  measures "d15" distance of L4 L6
  measures "d16" distance of L5 L7
extrude "Extrude3" add sketch "Sketch4" against normal blind 2 contours L0 L4 L5 L6 L7 bodies 1
sketch "Sketch5" plane through (-30.55, 0, 0) normal (-1, 0, 0) x (0, -1, 0)
  line L0 (-57, 0) -> (0, 0)
  line L1 (0, 0) -> (0, 20)
  line L2 (0, 20) -> (-57, 20)
  line L3 (-57, 20) -> (-57, 0)
  line L4 (0, 0) -> (-20, 0)
  line L5 (-20, 0) -> (-20, -4)
  line L6 (-20, -4) -> (0, -4)
  line L7 (0, -4) -> (0, 0)
  dimension "d19" = 4
  dimension "d20" = 20
  constraint horizontal L4
  constraint vertical L5
  constraint horizontal L6
  constraint vertical L7
  constraint coincident L0.end L1.start
  measures "d19" distance of L4 L6
  measures "d20" distance of L5 L7
extrude "Extrude4" add sketch "Sketch5" against normal blind 2 contours L0 L4 L5 L6 L7 bodies 1
sketch "Sketch6" plane through (0, 0, 0) normal (0, -1, 0) x (1, 0, 0)
  line L0 (30.55, -4) -> (30.55, 20)
  line L1 (30.55, 20) -> (28.55, 20)
  line L2 (28.55, 20) -> (28.55, -4)
  line L3 (28.55, -4) -> (30.55, -4)
  line L4 (28.55, -4) -> (40.55, -4)
  line L5 (40.55, -4) -> (40.55, -14)
  line L6 (40.55, -14) -> (28.55, -14)
  line L7 (28.55, -14) -> (28.55, -4)
  line L8 (-28.55, -4) -> (-40.55, -4)
  line L9 (-40.55, -4) -> (-40.55, -14)
  line L10 (-40.55, -14) -> (-28.55, -14)
  line L11 (-28.55, -14) -> (-28.55, -4)
  dimension "d23" = 57.1
  dimension "d24" = 12
  dimension "d25" = 10
  dimension "d26" = 12
  constraint horizontal L4
  constraint vertical L5
  constraint horizontal L6
  constraint vertical L7
  constraint coincident L2.end L3.start
  constraint horizontal L8
  constraint vertical L9
  constraint horizontal L10
  constraint vertical L11
  constraint horizontal L6.end L10.end
  constraint horizontal L2.end L8.start
  measures "d23" distance of L2.end L8.start
  measures "d24" distance of L5 L7
  measures "d25" distance of L4 L6
  measures "d26" distance of L9 L11
extrude "Extrude5" add sketch "Sketch6" against normal blind 20 contours L3 L4 L5 L6 L7 | L8 L9 L10 L11 bodies 1
sketch "Sketch7" plane through (0, 0, -4) normal (0, 0, 1) x (-1, 0, 0)
  line L0 (-30.55, -20) -> (-30.55, 0)
  line L1 (-30.55, 0) -> (-40.55, 0)
  line L2 (-40.55, 0) -> (-40.55, -20)
  line L3 (-40.55, -20) -> (-30.55, -20)
  line L4 (40.55, 0) -> (40.55, -20)
  point P0 (-34.75, -10)
  point P1 (34.75, -10)
  dimension "d29" = 5.8
  dimension "d30" = 5.8
  dimension "d31" = 10
  constraint horizontal P0 P1
  measures "d29" distance of L2 P0
  measures "d30" distance of P1 L4
  measures "d31" distance of L1 P0
hole "Hole1" at (34.75, 10, -4) at (-34.75, 10, -4) direction (0, 0, -1) diameter 5.3 depth 20 tip angle 180 counterbore diameter 10 counterbore depth 5 bodies 1
fillet "Fillet1" radius 2 2 edges at (40.55, 20, -9) (-40.55, 20, -9) on bodies 1
fillet "Fillet2" radius 2 4 edges at (30.55, 57, 10) (-30.55, 57, 10) (29.55, 20, 0) (-29.55, 20, 0) on bodies 1